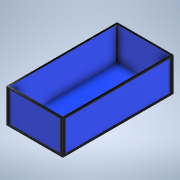
# Autodesk Inventor part: CustomAquariumsTank
Saved by Autodesk Inventor 2022 (Build 260153000, 153)
## iProperties
Created: 2021-06-23
Part Number: CustomAquariumsTank
Material: Generic
Document SubType Name: Modeling
Designer: jamieson-bl
Density: 1 g/cm^3
Appearance: Default
Author: jamieson-bl
Autodesk Inventor part; units mm, degrees
ref_plane "YZ Plane" through (0, 0, 0) normal (1, 0, 0) x (0, 1, 0)
ref_plane "XZ Plane" through (0, 0, 0) normal (0, 1, 0) x (-1, 0, 0)
ref_plane "XY Plane" through (0, 0, 0) normal (0, 0, 1) x (1, 0, 0)
sketch "Sketch1" plane through (0, 0, 0) normal (0, 1, 0) x (-1, 0, 0)
  line L0 (-762, -1524) -> (762, -1524)
  line L1 (762, -1524) -> (762, 1524)
  line L2 (762, 1524) -> (-762, 1524)
  line L3 (-762, 1524) -> (-762, -1524)
  line L4 (-762, -1524) -> (762, 1524) construction
  line L5 (762, -1524) -> (-762, 1524) construction
  point P0 (0, 0)
  dimension "d0" = 1524
  dimension "d1" = 3048
  constraints: 12 end point, 2 midpoint, 2 parallel, 1 horizontal, 1 perpendicular
  measures "d0" distance of L2.end L1.end
  measures "d1" distance of L1.end L0.end
extrude "Extrusion1" add sketch "Sketch1" along normal blind 914.4
sketch "Sketch2" plane through (0, 914.4, 0) normal (0, 1, 0) x (1, 0, 0)
  line L0 (742.95, 1504.95) -> (-742.95, 1504.95)
  line L1 (-742.95, 1504.95) -> (-742.95, -1504.95)
  line L2 (-742.95, -1504.95) -> (742.95, -1504.95)
  line L3 (742.95, -1504.95) -> (742.95, 1504.95)
  line L4 (742.95, 1504.95) -> (-742.95, -1504.95) construction
  line L5 (-742.95, 1504.95) -> (742.95, -1504.95) construction
  point P0 (0, 0)
  dimension "d4" = 1485.9
  dimension "d5" = 3009.9
  constraints: 12 end point, 2 midpoint, 2 parallel, 1 horizontal, 1 perpendicular
  measures "d4" distance of L2.end L1.end
  measures "d5" distance of L1.end L0.end
extrude "Extrusion2" cut sketch "Sketch2" against normal blind 895.35
sketch "Sketch3" plane through (0, 914.4, 0) normal (0, 1, 0) x (1, 0, 0)
  line L0 (793.75, 1555.75) -> (-793.75, 1555.75)
  line L1 (-793.75, 1555.75) -> (-793.75, -1555.75)
  line L2 (-793.75, -1555.75) -> (793.75, -1555.75)
  line L3 (793.75, -1555.75) -> (793.75, 1555.75)
  line L4 (793.75, 1555.75) -> (-793.75, -1555.75) construction
  line L5 (-793.75, 1555.75) -> (793.75, -1555.75) construction
  line L6 (-742.95, -1504.95) -> (-742.95, 1504.95) projected
  line L7 (742.95, 1504.95) -> (-742.95, 1504.95)
  line L8 (-742.95, 1504.95) -> (-742.95, -1504.95)
  line L9 (-742.95, -1504.95) -> (742.95, -1504.95)
  line L10 (742.95, -1504.95) -> (742.95, 1504.95)
  line L11 (742.95, 1504.95) -> (-742.95, -1504.95) construction
  line L12 (-742.95, 1504.95) -> (742.95, -1504.95) construction
  point P0 (0, 0)
  dimension "d8" = 1587.5
  dimension "d9" = 3111.5
  constraints: 24 end point, 4 midpoint, 4 parallel, 2 horizontal, 2 perpendicular
  measures "d8" distance of L2.end L1.end
  measures "d9" distance of L1.end L0.end
extrude "Extrusion3" add sketch "Sketch3" along normal blind 31.75
pattern_linear "Rectangular Pattern1" count 2 spacing 914.4 along (0, -1, 0) of "Extrusion3"
sketch "Sketch4" plane through (-793.75, 31.75, 1555.75) normal (0, 1, 0) x (1, 0, 0)
  line L0 (0, 0) -> (1587.5, 0) projected
  line L1 (1587.5, 0) -> (1587.5, 76.2)
  line L2 (1587.5, 0) -> (1587.5, 3111.5) projected
  line L3 (1587.5, 76.2) -> (1536.7, 76.2)
  line L4 (1536.7, 3060.7) -> (1536.7, 50.8) projected
  line L5 (1536.7, 76.2) -> (1536.7, 50.8)
  line L6 (1536.7, 50.8) -> (1511.3, 50.8)
  line L7 (1536.7, 50.8) -> (50.8, 50.8) projected
  line L8 (1511.3, 50.8) -> (1511.3, 0)
  line L9 (1511.3, 0) -> (1587.5, 0)
  point P0 (793.75, 1555.75)
  dimension "d15" = 76.2
  dimension "d16" = 50.8
  dimension "d17" = 25.4
  dimension "d23" = 25.4
  dimension "d24" = 50.8
  dimension "d25" = 76.2
  constraints: 12 end point, 3 point on line, 2 perpendicular, 1 collinear
  measures "d15" distance of L0.end L1.end
  measures "d16" distance of L1.end L3.end
  measures "d17" distance of L4.end L6.end
  measures "d23" distance of L3.end L4.end
  measures "d24" distance between parallel lines of L0 L7
  measures "d25" distance between parallel lines of L1 L8
extrude "Extrusion4" add sketch "Sketch4" along normal blind 889
pattern_linear "Rectangular Pattern2" count 2 spacing 1511.3 along (-1, 0, 0) of "Extrusion4"
mirror "Mirror1" about plane through (0, 0, 0) normal (0, 0, 1) of "Extrusion4", "Rectangular Pattern2"
body "Solid1"
